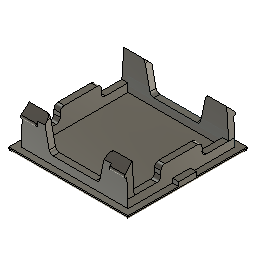
schaltwand-leuchtmelder-abdeckung v4 (Autodesk Fusion 360 design; units mm, degrees)
Autodesk Fusion 360 part; units mm, degrees
sketch "Skizze1" plane through (0, 0, 0) normal (0, 0, 1) x (1, 0, 0)
  line L0 (0, 0) -> (29, 0)
  line L1 (29, 0) -> (29, 29)
  line L2 (29, 29) -> (0, 29)
  line L3 (0, 29) -> (0, 0)
  dimension "d1" = 29
  dimension "d2" = 29
  constraint horizontal L0
  constraint vertical L1
  constraint horizontal L2
  constraint vertical L3
  constraint coincident L0.start L3.end
  measures "d1" distance of L0.start L0.end
  measures "d2" distance of L0.start L2.end
extrude "Extrusion1" add sketch "Skizze1" along normal blind 1
fillet "Abrundung1" radius 0.7 4 edges at (14.5, 0, 0) (29, 14.5, 0) (14.5, 29, 0) (0, 14.5, 0)
sketch "Skizze2" plane through (0, 0, 1) normal (0, 0, 1) x (-1, 0, 0)
  line L0 (0, -29) -> (0, 0)
  line L1 (0, 0) -> (-29, 0)
  line L2 (-29, 0) -> (-29, -29)
  line L3 (-29, -29) -> (0, -29)
  line L4 (-1.5, -27.5) -> (-27.5, -27.5)
  line L5 (-27.5, -27.5) -> (-27.5, -1.5)
  line L6 (-27.5, -1.5) -> (-1.5, -1.5)
  line L7 (-1.5, -1.5) -> (-1.5, -27.5)
  line L8 (-26, -26) -> (-26, -3)
  line L9 (-26, -3) -> (-3, -3)
  line L10 (-3, -3) -> (-3, -26)
  line L11 (-3, -26) -> (-26, -26)
  dimension "d7" = 26
  dimension "d8" = 26
  dimension "d9" = 29
  dimension "d10" = 1.5
  dimension "d11" = 1.5
  dimension "d12" = 1.5
  constraint horizontal L4
  constraint vertical L5
  constraint horizontal L6
  constraint vertical L7
  measures "d7" distance of L4.start L4.end
  measures "d8" distance of L4.start L6.end
  measures "d9" distance of L0 L1.end
  measures "d10" distance of L0 L7
  measures "d11" distance of L3 L4
extrude "Extrusion2" add sketch "Skizze2" along normal blind 2 contours L4 L5 L6 L7
sketch "Skizze3" plane through (1.5, 0, 0) normal (-1, 0, 0) x (0, -1, 0)
  line L0 (-27.5, 1) -> (-1.5, 1)
  line L1 (-1.5, 1) -> (-1.5, 3)
  line L2 (-1.5, 3) -> (-27.5, 3)
  line L3 (-27.5, 3) -> (-27.5, 1)
  line L4 (-9.5, 4) -> (-9.5, 5)
  line L5 (-10.5, 6) -> (-18.5, 6)
  line L6 (-19.5, 5) -> (-19.5, 4)
  line L7 (-8.5, 3) -> (-1.5, 3)
  line L8 (-27.5, 3) -> (-20.5, 3)
  arc A0 (-20.5, 3) -> (-19.5, 4) centre (-20.5, 4) ccw
  line L9 (-9.5, 3) -> (-1.5, 3)
  arc A1 (-9.5, 4) -> (-8.5, 3) centre (-8.5, 4) ccw
  arc A2 (-18.5, 6) -> (-19.5, 5) centre (-18.5, 5) ccw
  arc A3 (-9.5, 5) -> (-10.5, 6) centre (-10.5, 5) ccw
  point P0 (-19.5, 3)
  point P1 (-19.5, 6)
  dimension "d15" = 10
  dimension "d16" = 3
  dimension "d17" = 26
  dimension "d18" = 8
  dimension "d19" = 1
  dimension "d20" = 1
  dimension "d21" = 1
  dimension "d22" = 1
  constraint vertical L4
  constraint horizontal L5
  constraint vertical L6
  constraint coincident L2 P0
  constraint coincident L1.end L2.start
  constraint perpendicular L1 L7
  constraint coincident L2.end L3.start
  constraint coincident P0 L8
  constraint coincident P0 L6
  constraint tangent L8 A0
  constraint tangent L6 A0
  constraint coincident L9.start L4
  constraint coincident L9.start L7
  constraint tangent L4 A1
  constraint tangent L7 A1
  constraint coincident P1 L6
  constraint coincident P1 L5
  constraint tangent L6 A2
  constraint tangent L5 A2
  constraint tangent L5 A3
  constraint tangent L4 A3
  measures "d15" distance of P0 L9.start
  measures "d16" distance of P0 P1
  measures "d17" distance of L1 L3
  measures "d18" distance of L1 L4
  measures "d19" radius of A0
  measures "d20" radius of A1
  measures "d21" radius of A2
  measures "d22" radius of A3
extrude "Extrusion3" add sketch "Skizze3" against normal up to surface (26 mm away) contours L2 L4 L5 L6 A0 L9 A1 A2 A3
extrude "Extrusion4" cut 1 faces at (10.6667, 18.3333, 1) along direction (0, 0, 1) blind 5
sketch "Skizze4" plane through (0, 27.5, 0) normal (0, 1, 0) x (-1, 0, 0)
  line L0 (-27.5, 1) -> (-1.5, 1)
  line L1 (-1.5, 1) -> (-1.5, 3)
  line L2 (-1.5, 3) -> (-27.5, 3)
  line L3 (-27.5, 3) -> (-27.5, 1)
sketch "Skizze5" plane through (0, 0, 1) normal (0, 0, 1) x (-1, 0, 0)
  line L0 (0, -29) -> (0, 0)
  line L1 (0, 0) -> (-29, 0)
  line L2 (-29, 0) -> (-29, -29)
  line L3 (-29, -29) -> (0, -29)
  line L4 (-1.5, -1.5) -> (-1.5, -27.5)
  line L5 (-1.5, -27.5) -> (-27.5, -27.5)
  line L6 (-27.5, -27.5) -> (-27.5, -1.5)
  line L7 (-27.5, -1.5) -> (-1.5, -1.5)
  line L8 (-27.5, -16.65) -> (-29, -16.65)
  line L9 (-29, -16.65) -> (-29, -12.35)
  line L10 (-29, -12.35) -> (-27.5, -12.35)
  line L11 (-27.5, -12.35) -> (-27.5, -16.65)
  line L12 (-27.5, -12.35) -> (0, -12.35) construction
  line L13 (0, -12.35) -> (-1.5, -12.35)
  line L14 (-1.5, -12.35) -> (-1.5, -16.65)
  line L15 (-1.5, -16.65) -> (0, -16.65)
  line L16 (0, -16.65) -> (0, -12.35)
  dimension "d27" = 4.3
  dimension "d28" = 29
  dimension "d29" = 12.35
  dimension "d30" = 4.3
  constraint horizontal L8
  constraint vertical L9
  constraint horizontal L10
  constraint vertical L11
  constraint coincident L6 L8.start
  constraint coincident L0 L12.end
  constraint perpendicular L0 L12
  constraint horizontal L13
  constraint vertical L14
  constraint horizontal L15
  constraint vertical L16
  constraint coincident L4 L14.end
  measures "d27" distance of L8.start L10.end
  measures "d28" distance of L1 L3
  measures "d29" distance of L1 L10
  measures "d30" distance of L12 L15
extrude "Extrusion5" add sketch "Skizze5" along normal blind 1 contours L0 L4 L13 L14 L15 L16 | L2 L6 L8 L9 L10 L11
sketch "Skizze6" plane through (0, 27.5, 0) normal (0, 1, 0) x (-1, 0, 0)
  line L0 (-27.5, 1) -> (-1.5, 1)
  line L1 (-1.5, 1) -> (-1.5, 3)
  line L2 (-1.5, 3) -> (-27.5, 3)
  line L3 (-27.5, 3) -> (-27.5, 1)
  line L4 (-29.2103, 10) -> (4.3331, 10) construction
  line L5 (-1.5, 3) -> (-27.5, 3)
  line L6 (-1.5, 3) -> (-1.5, 10) construction
  line L7 (-1.5, 3) -> (-2, 10)
  line L8 (-14.5, 3) -> (-14.5, 12.4711) construction
  line L9 (-2, 10) -> (-6.1916, 10)
  line L10 (-7.1694, 9.2095) -> (-8.3306, 3.7905)
  line L11 (-1.5, 3) -> (-14.5, 3)
  arc A0 (-9.3084, 3) -> (-8.3306, 3.7905) centre (-9.3084, 4) ccw
  arc A1 (-6.1916, 10) -> (-7.1694, 9.2095) centre (-6.1916, 9) ccw
  line L12 (-21.8306, 9.2095) -> (-20.6694, 3.7905)
  arc A2 (-21.8306, 9.2095) -> (-22.8084, 10) centre (-22.8084, 9) ccw
  line L13 (-27, 10) -> (-22.8084, 10)
  line L14 (-27.5, 3) -> (-27, 10)
  arc A3 (-20.6694, 3.7905) -> (-19.6916, 3) centre (-19.6916, 4) ccw
  line L15 (-27.5, 3) -> (-14.5, 3)
  point P0 (-7, 10)
  dimension "d33" = 7
  dimension "d34" = 0.5
  dimension "d36" = 5
  dimension "d37" = 1
  dimension "d38" = 1
  constraint horizontal L4
  constraint coincident L1.end L2.start
  constraint coincident L4 L6.end
  constraint perpendicular L4 L6
  constraint coincident L4 L7.end
  constraint midpoint L5 L8.start
  constraint perpendicular L4 L8
  constraint perpendicular L1 L11
  constraint parallel L4 L9
  constraint tangent L11 A0
  constraint tangent L10 A0
  constraint coincident P0 L10
  constraint coincident P0 L9
  constraint tangent L10 A1
  constraint tangent L9 A1
  constraint symmetric L1.end L8 L2.end
  constraint symmetric L7.end L8 L13.start
  constraint symmetric L11.end L8 L15.end
  constraint symmetric L8 A0.start A3.end
  constraint symmetric L8 L10.end L12.end
  constraint symmetric L8 A0 A3
  constraint symmetric L8 L10.start L12.start
  constraint symmetric L8 L9.end A2.end
  constraint symmetric L8 A1 A2
  measures "d33" distance of L4 L5
  measures "d34" distance of L6 L7.end
  measures "d36" distance of L7.end P0
  measures "d37" radius of A0
  measures "d38" radius of A1
extrude "Extrusion6" add sketch "Skizze6" against normal up to surface (1.5 mm away) contours L2 L5 L12 A2 L13 L14 A3 L15 | L2 L5 L7 L9 L10 L11 A0 A1
sketch "Skizze7" plane through (27.5, 0, 0) normal (1, 0, 0) x (0, 1, 0)
  line L0 (16.65, 2) -> (16.65, 1)
  line L1 (16.65, 1) -> (27.5, 1)
  line L2 (27.5, 1) -> (27.5, 3)
  line L3 (27.5, 3) -> (26, 3)
  line L4 (26, 3) -> (20.5, 3)
  arc A0 (19.5, 4) -> (20.5, 3) centre (20.5, 4) ccw
  line L5 (19.5, 4) -> (19.5, 5)
  arc A1 (19.5, 5) -> (18.5, 6) centre (18.5, 5) ccw
  line L6 (18.5, 6) -> (10.5, 6)
  arc A2 (10.5, 6) -> (9.5, 5) centre (10.5, 5) ccw
  line L7 (9.5, 5) -> (9.5, 4)
  arc A3 (8.5, 3) -> (9.5, 4) centre (8.5, 4) ccw
  line L8 (8.5, 3) -> (1.5, 3)
  line L9 (1.5, 3) -> (1.5, 1)
  line L10 (1.5, 1) -> (12.35, 1)
  line L11 (12.35, 1) -> (12.35, 2)
  line L12 (12.35, 2) -> (16.65, 2)
  line L13 (26, 10) -> (26, 3)
  line L14 (26, 3) -> (27.5, 3)
  line L15 (27.5, 3) -> (27.5, 10)
  line L16 (27.5, 10) -> (26, 10)
  line L17 (26, 10) -> (27.6131, 8.3869)
  line L18 (26, 10) -> (28.2813, 10) construction
  dimension "d41" = 45
  constraint horizontal L18
  constraint coincident L13.start L16.end
  measures "d41" angle of L17 L18
extrude "Extrusion7" cut sketch "Skizze7" against normal blind 29 contours L15 L16 L17
sketch "Skizze9" plane through (27.5, 0, 0) normal (1, 0, 0) x (0, 1, 0)
  line L0 (16.65, 2) -> (16.65, 1)
  line L1 (16.65, 1) -> (27.5, 1)
  line L2 (27.5, 1) -> (27.5, 3)
  line L3 (27.5, 3) -> (26, 3)
  line L4 (26, 3) -> (20.5, 3)
  arc A0 (19.5, 4) -> (20.5, 3) centre (20.5, 4) ccw
  line L5 (19.5, 4) -> (19.5, 5)
  arc A1 (19.5, 5) -> (18.5, 6) centre (18.5, 5) ccw
  line L6 (18.5, 6) -> (10.5, 6)
  arc A2 (10.5, 6) -> (9.5, 5) centre (10.5, 5) ccw
  line L7 (9.5, 5) -> (9.5, 4)
  arc A3 (8.5, 3) -> (9.5, 4) centre (8.5, 4) ccw
  line L8 (8.5, 3) -> (1.5, 3)
  line L9 (1.5, 3) -> (1.5, 1)
  line L10 (1.5, 1) -> (12.35, 1)
  line L11 (12.35, 1) -> (12.35, 2)
  line L12 (12.35, 2) -> (16.65, 2)
  line L13 (27.5, 8.5) -> (26, 10)
  line L14 (26, 10) -> (26, 3)
  line L15 (26, 3) -> (27.5, 3)
  line L16 (27.5, 3) -> (27.5, 8.5)
  line L17 (27.5, 8.5) -> (27.8536, 8.1464)
  arc A4 (27.5, 7.2929) -> (27.8536, 8.1464) centre (27.5, 7.7929) ccw
  dimension "d44" = 1
  constraint parallel L13 L17
  constraint coincident L16 A4.centre
  constraint tangent L17 A4
  constraint coincident L16 A4.start
  measures "d44" diameter of A4
extrude "Extrusion8" add sketch "Skizze9" against normal up to surface (26 mm away) contours L16 L17 A4
sketch "Skizze10" plane through (0, 27.5, 0) normal (0, 1, 0) x (-1, 0, 0)
  line L0 (-21.4199, 7.2929) -> (-27.1934, 7.2929)
  line L1 (-27.1934, 7.2929) -> (-27.5, 3)
  line L2 (-27.5, 3) -> (-27.5, 1)
  line L3 (-27.5, 1) -> (-1.5, 1)
  line L4 (-1.5, 1) -> (-1.5, 3)
  line L5 (-1.5, 3) -> (-1.8066, 7.2929)
  line L6 (-1.8066, 7.2929) -> (-7.5801, 7.2929)
  line L7 (-7.5801, 7.2929) -> (-8.3306, 3.7905)
  arc A0 (-9.3084, 3) -> (-8.3306, 3.7905) centre (-9.3084, 4) ccw
  line L8 (-9.3084, 3) -> (-19.6916, 3)
  arc A1 (-20.6694, 3.7905) -> (-19.6916, 3) centre (-19.6916, 4) ccw
  line L9 (-20.6694, 3.7905) -> (-21.4199, 7.2929)
  line L10 (-7.3214, 8.5) -> (-7.1694, 9.2095)
  line L11 (-21.8306, 9.2095) -> (-21.6786, 8.5)
  line L12 (-27.1071, 8.5) -> (-27, 10)
  line L13 (-2, 10) -> (-1.8929, 8.5)
  line L14 (-1.8929, 8.5) -> (-1.8066, 7.2929)
  line L15 (-7.3214, 8.5) -> (-7.5801, 7.2929)
  line L16 (-27.1071, 8.5) -> (-27.1934, 7.2929)
  line L17 (-21.6786, 8.5) -> (-21.4199, 7.2929)
  line L18 (-1.5, 8.1464) -> (-1.5, 7.2929)
  line L19 (-1.5, 8.1464) -> (-27.5, 8.1464)
  line L20 (-27.5, 8.1464) -> (-27.5, 7.2929)
  line L21 (-27.5, 7.2929) -> (-27.1934, 7.2929)
  line L22 (-27.1934, 7.2929) -> (-21.4199, 7.2929)
  line L23 (-21.4199, 7.2929) -> (-7.5801, 7.2929)
  line L24 (-7.5801, 7.2929) -> (-1.8066, 7.2929)
  line L25 (-1.8066, 7.2929) -> (-1.5, 7.2929)
  line L26 (-27, 10) -> (-27.1071, 8.5)
  line L27 (-27.1071, 8.5) -> (-27.5, 8.5)
  line L28 (-27.5, 8.5) -> (-27.5, 8.1464)
  line L29 (-27.5, 8.1464) -> (-1.5, 8.1464)
  line L30 (-1.5, 8.1464) -> (-1.5, 8.5)
  line L31 (-1.5, 8.5) -> (-1.8929, 8.5)
  line L32 (-1.8929, 8.5) -> (-2, 10)
  line L33 (-2, 10) -> (-6.1916, 10)
  arc A2 (-6.1916, 10) -> (-7.1694, 9.2095) centre (-6.1916, 9) ccw
  line L34 (-7.1694, 9.2095) -> (-7.3214, 8.5)
  line L35 (-7.3214, 8.5) -> (-21.6786, 8.5)
  line L36 (-21.6786, 8.5) -> (-21.8306, 9.2095)
  arc A3 (-21.8306, 9.2095) -> (-22.8084, 10) centre (-22.8084, 9) ccw
  line L37 (-22.8084, 10) -> (-27, 10)
  line L38 (-27.5, 8.5) -> (-1.5, 8.5)
  line L39 (-1.5, 8.5) -> (-1.5, 7.2929)
  line L40 (-1.5, 7.2929) -> (-27.5, 7.2929)
  line L41 (-27.5, 7.2929) -> (-27.5, 8.5)
  constraint coincident L13.end L14.start
  constraint coincident L5.end L6.start
  constraint coincident L10.start L15.start
  constraint coincident L6.end L7.start
  constraint coincident L12.start L16.start
  constraint coincident L0.end L1.start
  constraint coincident L11.end L17.start
  constraint coincident L0.start L9.end
  constraint horizontal L38
  constraint vertical L39
  constraint horizontal L40
  constraint vertical L41
  constraint coincident L18.end L25.end
  constraint coincident L27.end L28.start
extrude "Extrusion9" cut sketch "Skizze10" along normal blind 1.5 contours L15 L17 L19 L23 L29 L40 | L16 L19 L20 L21 L29 L40 L41 | L15 L17 L19 L29 L35 L38 | L16 L19 L27 L28 L29 L38 L41 | L14 L18 L19 L25 L29 L39 L40 | L14 L19 L29 L30 L31 L38 L39
sketch "Skizze11" plane through (0, 0, 1) normal (0, 0, 1) x (-1, 0, 0)
  line L0 (-27.5, -16.65) -> (-29, -16.65)
  line L1 (-29, -16.65) -> (-29, -29)
  line L2 (-29, -29) -> (0, -29)
  line L3 (0, -29) -> (0, -16.65)
  line L4 (0, -16.65) -> (-1.5, -16.65)
  line L5 (-1.5, -16.65) -> (-1.5, -27.5)
  line L6 (-1.5, -27.5) -> (-27.5, -27.5)
  line L7 (-27.5, -27.5) -> (-27.5, -16.65)
  ellipse E0 centre (-7.473, -27.5) end of major axis (-7.473, -27) minor radius 0.1071 (-7.5801, -27.5) -> (-7.3972, -27.8536) ccw
  ellipse E1 centre (-21.527, -27.5) end of major axis (-21.527, -28) minor radius 0.1071 (-21.6028, -27.8536) -> (-21.4199, -27.5) ccw
  ellipse E2 centre (-27.1577, -27.5) end of major axis (-27.1577, -27) minor radius 0.0357 (-27.1934, -27.5) -> (-27.1324, -27.8536) ccw
  ellipse E3 centre (-1.8423, -27.5) end of major axis (-1.8423, -28) minor radius 0.0357 (-1.8676, -27.8536) -> (-1.8066, -27.5) ccw
  line L8 (-7.5801, -27.5) -> (-5.5801, -27.5)
  line L9 (-5.5801, -27.5) -> (-5.5801, -29)
  line L10 (-5.5801, -29) -> (-7.5801, -29)
  line L11 (-7.5801, -29) -> (-7.5801, -27.5)
  line L12 (-21.4199, -27.5) -> (-23.4199, -27.5)
  line L13 (-23.4199, -27.5) -> (-23.4199, -29)
  line L14 (-23.4199, -29) -> (-21.4199, -29)
  line L15 (-21.4199, -29) -> (-21.4199, -27.5)
  dimension "d49" = 2
  dimension "d50" = 2
  constraint horizontal L8
  constraint vertical L9
  constraint horizontal L10
  constraint vertical L11
  constraint coincident L8.start L11.end
  constraint horizontal L12
  constraint vertical L13
  constraint horizontal L14
  constraint vertical L15
  constraint coincident L12.start L15.end
  measures "d49" distance of L8.start L8.end
  measures "d50" distance of L12.start L12.end
extrude "Extrusion10" cut sketch "Skizze11" along normal blind 12 contours L2 L6 L12 L13 L14 L15 | L2 L6 L8 L9 L10 L11
sketch "Skizze12" plane through (0, 0, 1) normal (0, 0, 1) x (-1, 0, 0)
  line L0 (-3, -3) -> (-26, -3)
  line L1 (-26, -3) -> (-26, -26)
  line L2 (-26, -26) -> (-3, -26)
  line L3 (-3, -26) -> (-3, -3)
  line L4 (-26, -14.5) -> (1.3472, -14.5)
  line L5 (-26, -14.5) -> (-29.3311, -14.5)
  line L6 (-29, -12.35) -> (-27.5, -12.35)
  line L7 (-27.5, -12.35) -> (-27.5, -1.5)
  line L8 (-27.5, -1.5) -> (-1.5, -1.5)
  line L9 (-1.5, -1.5) -> (-1.5, -12.35)
  line L10 (-1.5, -12.35) -> (0, -12.35)
  line L11 (0, -12.35) -> (0, 0)
  line L12 (0, 0) -> (-29, 0)
  line L13 (-29, 0) -> (-29, -12.35)
  line L14 (-29, -12.35) -> (-29, -16.65)
  line L15 (0, -16.65) -> (0, -12.35)
  line L16 (0, -14.5) -> (-29, -14.5)
  line L17 (-29, -14.5) -> (-29, 0)
  line L18 (-29, 0) -> (0, 0)
  line L19 (0, 0) -> (0, -14.5)
  constraint midpoint L1 L4.start
  constraint perpendicular L3 L4
  constraint perpendicular L1 L5
  constraint horizontal L16
  constraint vertical L17
  constraint horizontal L18
  constraint vertical L19
  constraint coincident L12.end L13.start
  constraint midpoint L15 L16.start
extrude "Extrusion11" cut sketch "Skizze12" along normal blind 8 and the other way blind 3 contours L0 L1 L3 L4 L16 | L0 L1 L3 L4 L5 L6 L7 L8 L9 L10 L14 L15 L16 L17 L19 | L6 L7 L8 L9 L10 L11 L12 L13 L17 L18 L19
mirror "Spiegeln1" about plane through (26, 14.5, 1) normal (0, -1, 0) of bodies 1 merged
equation "d10 = ( d9 - d7 ) / 2"
equation "d11 = d10"
equation "d18 = ( d17 - d15 ) / 2"
equation "d29 = ( d28 - d27 ) / 2"
equation "d30 = d27"
